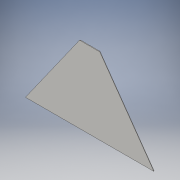
# Autodesk Inventor part: Nexus 7 3D hologram frame
Saved by Autodesk Inventor 2016 (Build 200138000, 138)
## iProperties
Created: 2017-08-31
Part Number: Nexus 7 3D hologram frame
Material: Generic
Document SubType Name: Modeling
Designer: student
Density: 1 g/cm^3
Appearance: Default
Author: student
Autodesk Inventor part; units mm, degrees
ref_plane "YZ Plane" through (0, 0, 0) normal (1, 0, 0) x (0, 1, 0)
ref_plane "XZ Plane" through (0, 0, 0) normal (0, 1, 0) x (-1, 0, 0)
ref_plane "XY Plane" through (0, 0, 0) normal (0, 0, 1) x (1, 0, 0)
sketch "Sketch1" plane through (0, 0, 0) normal (0, 0, 1) x (1, 0, 0)
  line L0 (-7.5, 28.2811) -> (7.5, 28.2811)
  line L1 (47.5, -28.285) -> (-47.5, -28.285)
  line L2 (7.5, 28.2811) -> (47.5, -28.285)
  line L3 (-7.5, 28.2811) -> (-47.5, -28.285)
  point P0 (0, 0)
  point P1 (0, 28.2811)
  point P2 (0, -28.285)
  dimension "d0" = 69.28
  dimension "d1" = 95
  dimension "d2" = 15
  dimension "d3" = 56.566
  dimension "d4" = 69.28
  constraints: 8 end point, 2 midpoint, 1 horizontal, 1 parallel, 1 vertical alignment
  measures "d0" distance of L0.end L1.start
  measures "d1" distance of L1.start L1.end
  measures "d2" distance of L0.start L0.end
  measures "d3" distance between parallel lines of L1 L0
  measures "d4" distance of L0.start L1.end
extrude "Extrusion1" add sketch "Sketch1" along normal blind 0.5
chamfer "Chamfer2" distance 0.5 angle 30 1 edges at (27.5, -0.002, 0) measured on face at (27.5, -0.002, 0.1)
chamfer "Chamfer3" distance 0.5 angle 30 1 edges at (-27.5, -0.002, 0) measured on face at (-27.5, -0.002, 0.1)
body "Solid1"
